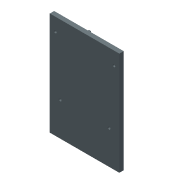
# Autodesk Inventor part: bas_plate
Saved by Autodesk Inventor 2022 (Build 260148000, 148)
## iProperties
Shininess: 64.0
Length Units: 11272
Angle Units: 11279
Time Units: 11290
Mass Units: 11286
Length Display Precision: 3
Angle Display Precision: 2
Created: 2002-04-25
Part Number: bas_plate
Document SubType Name: Modeling
Designer: Administrator
Density: 1 g/cm^3
Material: Generic
Appearance: Blue Grey (Light)
Density: 0.0
Volumn: 0.0
Area: 0.0
PropertySet Name: Model Information
Control State: 0
Master: False
Checked Out: False
Author: Administrator
Autodesk Inventor part; units mm, degrees
ref_plane "YZ Plane" through (0, 0, 0) normal (1, 0, 0) x (0, 1, 0)
ref_plane "XZ Plane" through (0, 0, 0) normal (0, 1, 0) x (-1, 0, 0)
ref_plane "XY Plane" through (0, 0, 0) normal (0, 0, 1) x (1, 0, 0)
sketch "Sketch1" plane through (0, 0, 0) normal (0, 0, 1) x (1, 0, 0)
  line L0 (-25.5474, 19.5864) -> (55.7326, 19.5864)
  line L1 (55.7326, 19.5864) -> (55.7326, -101.0636)
  line L2 (55.7326, -101.0636) -> (-25.5474, -101.0636)
  line L3 (-25.5474, -101.0636) -> (-25.5474, 19.5864)
  dimension "d0" = 81.28
  dimension "d1" = 120.65
  constraints: 8 end point, 2 parallel, 1 horizontal, 1 perpendicular
  measures "d0" distance of L0.start L0.end
  measures "d1" distance of L2.end L0.start
extrude "Extrusion1" add sketch "Sketch1" along normal blind 5.08
sketch "Sketch2" plane through (0, 0, 5.08) normal (0, 0, 1) x (1, 0, 0)
  line L0 (55.7326, 19.5864) -> (55.7326, -101.0636) projected
  line L1 (-25.5474, 19.5864) -> (55.7326, 19.5864) projected
  line L2 (-25.5474, -101.0636) -> (-25.5474, 19.5864) projected
  line L3 (55.7326, -101.0636) -> (-25.5474, -101.0636) projected
  line L4 (-19.1974, 4.3464) -> (49.3826, 4.3464)
  line L5 (49.3826, 4.3464) -> (43.6676, -61.6936)
  line L6 (43.6676, -61.6936) -> (-13.4824, -61.6936)
  line L7 (-13.4824, -61.6936) -> (-19.1974, 4.3464)
  circle A0 centre (15.0926, 4.3464) radius 40.64 construction
  circle A1 centre (15.0926, 4.3464) radius 34.29 construction
  circle A2 centre (15.0926, -61.6936) radius 28.575 construction
  dimension "d4" = 57.15
  dimension "d5" = 68.58
  dimension "d6" = 15.24
  dimension "d7" = 66.04
  constraints: 8 end point, 4 point on circle, 3 centre point, 2 midpoint, 2 tangent, 1 coincident, 1 horizontal, 1 parallel, 1 vertical alignment
  measures "d4" distance of L5.end L6.end
  measures "d5" distance of L4.start L4.end
  measures "d6" distance between parallel lines of L4 L1
  measures "d7" vertical distance of L6.end L4.start
hole "Hole1" at (-19.1974, 4.3464, 5.08) at (49.3826, 4.3464, 5.08) at (43.6676, -61.6936, 5.08) at (-13.4824, -61.6936, 5.08) direction (0, 0, -1) diameter 3.175 end through all
sketch "Sketch4" plane through (-25.5474, 19.5864, 0) normal (0, 1, 0) x (1, 0, 0)
  line L0 (81.28, 0) -> (81.28, -5.08) projected
  line L1 (0, 0) -> (81.28, 0) projected
  line L2 (0, 0) -> (0, -5.08) projected
  line L3 (39.37, 0) -> (41.91, 0)
  line L4 (41.91, 0) -> (41.91, 1.27)
  line L5 (41.91, 1.27) -> (39.37, 1.27)
  line L6 (39.37, 1.27) -> (39.37, 0)
  circle A0 centre (40.64, 0.4048) radius 1.27 construction
  circle A1 centre (40.64, 0.4048) radius 40.64 construction
  dimension "d15" = 2.54
  dimension "d16" = 1.27
  constraints: 8 end point, 4 tangent, 2 centre point, 2 parallel, 1 coincident, 1 horizontal, 1 perpendicular, 1 point on line
  measures "d15" distance of L4.end L5.end
  measures "d16" distance of L3.end L4.end
extrude "Extrusion2" add sketch "Sketch4" against normal blind 12.7
sketch "Sketch5" plane through (-25.5474, 6.8864, 0) normal (0, -1, 0) x (1, 0, 0)
  line L0 (41.91, 0) -> (41.91, -1.27) projected
  line L1 (39.37, 0) -> (41.91, 0) projected
  line L2 (39.37, -1.27) -> (39.37, 0) projected
  line L3 (41.91, -1.27) -> (39.37, -1.27) projected
  line L4 (27.94, 0) -> (53.34, 0)
  line L5 (53.34, 0) -> (53.34, -1.27)
  line L6 (53.34, -1.27) -> (27.94, -1.27)
  line L7 (27.94, -1.27) -> (27.94, 0)
  circle A0 centre (40.64, -8.0178) radius 1.27 construction
  circle A1 centre (40.64, -8.0178) radius 12.7 construction
  dimension "d19" = 25.4
  constraints: 8 end point, 4 tangent, 2 centre point, 2 collinear, 2 parallel, 1 coincident, 1 horizontal, 1 perpendicular
  measures "d19" distance of L5.end L6.end
extrude "Extrusion3" add sketch "Sketch5" against normal blind 2.54
sketch "Sketch7" plane through (0, 0, 0) normal (0, 0, -1) x (-1, 0, 0)
  line L0 (-55.7326, 19.5864) -> (-55.7326, -101.0636) projected
  line L1 (25.5474, -101.0636) -> (25.5474, 19.5864) projected
  circle A0 centre (13.4824, -61.6936) radius 1.5875 projected
  circle A1 centre (-5.5676, -86.3316) radius 5.08
  circle A2 centre (-5.5676, -86.3316) radius 1.905
  circle A3 centre (-24.6176, -86.3316) radius 5.08
  circle A4 centre (-24.6176, -86.3316) radius 1.905
  circle A5 centre (-15.0926, -74.2033) radius 15.4215 construction
  circle A6 centre (-15.0926, -74.2033) radius 40.64 construction
  dimension "d26" = 19.05
  dimension "d27" = 24.638
  dimension "d28" = 3.81
  dimension "d29" = 10.16
  constraints: 6 centre point, 3 coincident, 2 equal radius, 2 point on circle, 2 tangent, 1 horizontal alignment
  measures "d26" distance of A3.centre A1.centre
  measures "d27" vertical distance of A2.centre A0.centre
  measures "d28" diameter of A2
  measures "d29" diameter of A1
extrude "Extrusion5" add sketch "Sketch7" along normal blind 7.62 contours A1 | A3
body "Solid1"
